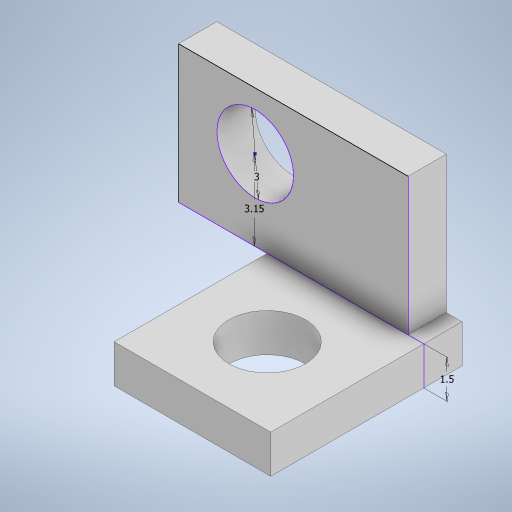
# Autodesk Inventor part: IMU_holder
Saved by Autodesk Inventor 2023.1 (Build 271208000, 208)
## iProperties
Created: 2023-01-31
Part Number: IMU_holder
Material: Generic
Document SubType Name: Modeling
Designer: Windows10
Density: 1 g/cm^3
Appearance: Default
Author: Windows10
Autodesk Inventor part; units mm, degrees
ref_plane "YZ Plane" through (0, 0, 0) normal (1, 0, 0) x (0, 1, 0)
ref_plane "XZ Plane" through (0, 0, 0) normal (0, 1, 0) x (-1, 0, 0)
ref_plane "XY Plane" through (0, 0, 0) normal (0, 0, 1) x (1, 0, 0)
sketch "Sketch1" plane through (0, 0, 0) normal (0, 0, 1) x (1, 0, 0)
  line L0 (0, 0) -> (9, 0)
  line L1 (9, 0) -> (9, -5.3835)
  line L2 (9, -5.3835) -> (0, -5.3835)
  line L3 (0, -5.3835) -> (0, 0)
  circle A0 centre (3, -2.2335) radius 1.5
  line L4 (3.4757, -5.3835) -> (9.6132, -5.3835)
  line L5 (9.6132, -5.3835) -> (9.6132, -6.8835)
  line L6 (9.6132, -6.8835) -> (3.4757, -6.8835)
  line L7 (3.4757, -6.8835) -> (3.4757, -5.3835)
  dimension "d0" = 3
  dimension "d1" = 3.15
  dimension "d8" = 1.5
  constraints: 16 end point, 4 parallel, 2 horizontal, 2 perpendicular, 1 centre point, 1 point on line
  measures "d0" diameter of A0
  measures "d1" distance from line of L2 A0.centre
  measures "d8" distance of L4.end L5.end
extrude "Extrusion1" add sketch "Sketch1" against normal blind 1.5
extrude "Extrusion2" add sketch "Sketch1" along normal blind 6 and the other way blind 1 contours L4 L5 L6 L7 L2
sketch "Sketch2" plane through (3.4757, -5.3835, 0) normal (0, 1, 0) x (1, 0, 0)
  circle A0 centre (3, -3) radius 1.5
  line L0 (1.0243, 0) -> (-1.9757, 0) projected
  line L1 (0, 0) -> (0, -6) projected
  point P0 (-3.4757, 0)
  point P1 (-0.4757, 0)
  dimension "d9" = 3
  dimension "d10" = 3
  dimension "d11" = 3
  constraints: 1 centre point
  measures "d9" diameter of A0
  measures "d10" distance from line of A0.centre L0
  measures "d11" distance from line of L1 A0.centre
extrude "Extrusion3" cut sketch "Sketch2" against normal blind 1.5
body "Solid1"
